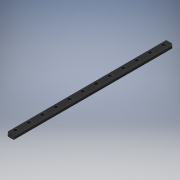
# Autodesk Inventor part: C-MLG9-235_r
Saved by Autodesk Inventor 2019 (Build 230136000, 136)
## iProperties
Created: 2023-08-25
Part Number: C-MLG9-235_r
Material: Generic
Catalog Web Link: www.cadenas.de
Description: C-MLG, C-MLGL, C-MLGB,C-GMLG, C-GMLGL_rail-Economy Miniature Liner guide - Standard type
Vendor: MISUMI
Document SubType Name: Modeling
Designer: psAdmin
Manufacturer: MISUMI
Mass: 11.5408 g
Surface Area: 89.2018 cm^2
Volume: 11.5408 cm^3
Density: 1 g/cm^3
Appearance: PSOLRGB-175-175-175
Category: PARTsolutions
Company: MISUMI
Title: C-MLG9-235
Author: Cadenas PARTsolutions
Comments: Economy Miniature Liner guide - Standard type
PSOL_IDENT_0: {$CADENAS_DATA/23d-libs/misumi/metric/06_linear_guides/c_mlg/c_mlg_rail.prj},209 {VTYP=3D},{NB=C-MLG
PSOL_IDENT_1: 9-235_r},{LINA=C-MLG9-235},{NN=C-MLG, C-MLGL, C-MLGB,C-GMLG, C-GMLGL_rail},{DATE=14.07.2023 05:43:34
PSOL_IDENT_2: },{GEOMDATE=01.12.2022 04:29:02},{VERSION=},{LINEID=20},{WBVAR=TS,ST,LT,L},{WBNUMERIC=L}  {NB=C-MLG9
PSOL_IDENT_3: -235_r},{LINA=C-MLG9-235},{KT=DUMMY},{PN=C-MLG9-235},{TS=},{ST=1},{LT=S},{LTALG='S', 'L Selectable T
PSOL_IDENT_4: ype', 'C', 'L Configurable Type'},{TYPE=C-MLG},{WR=9},{L=235},{LALG=[35,55,75,95,115,135,155,175,195
PSOL_IDENT_5: ,215,235,255,275]},{LALG1=[35,55,75,95,115,135,155,175,195,215,235,255,275]},{LALG2=[36:54/1],[56:74
PSOL_IDENT_6: /1],[76:94/1],[96:114/1],[116:134/1],[136:154/1],[156:174/1],[176:194/1],[196:214/1],[216:234/1],[23
PSOL_IDENT_7: 6:254/1],[256:274/1],[276:355/1]},{H=10},{H1=2.0},{N=5.5},{W=20},{B=15},{B1=2.5},{C=10},{L1=18.9},{L
PSOL_IDENT_8: 2=29.60},{GNN=Dia.1.4},{M=3},{LL=3.0},{ML=M3x3},{H2=1.8},{HRR=6.5},{D=6.0},{HH=3.5},{DD=3.5},{P=20},
PSOL_IDENT_9: {M1=12},{E=7.5},{NA=11},{R=1.00},{R1=0.400},{C1=0.30},{WR1=0.4},{WR2=0.92},{WR3=0.38},{HR1=4.5},{L3D=
PSOL_IDENT_10: 235.0},{LALG3=[35:355/1]}
NB: C-MLG9-235_r
NN: C-MLG, C-MLGL, C-MLGB,C-GMLG, C-GMLGL_rail
NT: Economy Miniature Liner guide - Standard type
NBSYN: $PN._r
LINA: C-MLG9-235
CATALOG: Misumi
PN: C-MLG9-235
TS: Assembly Products
ST: No Surface Treatment
LT: L Selectable Type
WR: 9
L: 235
H: 10
H1: 2
N: 5.5
W: 20
B: 15
B1: 2.5
C: 10
L1: 18.9
L2: 29.6
GNN: Dia.1.4
ML: M3x3
H2: 1.8
HRR: 6.5
D: 6
HH: 3.5
DD: 3.5
P: 20
E: 7.5
SUPPLIER: MISUMI
ARTICLENO: C-MLG9-235_r
BOMINFO: C-MLG9-235
CREATOR: CADENAS GmbH
Autodesk Inventor part; units mm, degrees
sketch "_____1" plane through (0, 0, 0) normal (0, 0, 1) x (1, 0, 0)
  line L0 (-4.5, 2.95) -> (-4.5, 2.1665)
  arc A0 (-3.9835, 1.65) -> (-4.5, 2.1665) centre (-4.9, 1.25) ccw
  line L1 (-3.9835, 1.65) -> (-3.6, 1.65)
  arc A1 (-3.6, 0.85) -> (-3.6, 1.65) centre (-3.6, 1.25) ccw
  line L2 (-3.6, 0.85) -> (-3.9835, 0.85)
  arc A2 (-4.5, 0.3335) -> (-3.9835, 0.85) centre (-4.9, 1.25) ccw
  line L3 (-4.5, 0.3335) -> (-4.5, -2.95)
  line L4 (-4.5, -2.95) -> (-4.2, -3.25)
  line L5 (-4.2, -3.25) -> (4.2, -3.25)
  line L6 (4.2, -3.25) -> (4.5, -2.95)
  line L7 (4.5, -2.95) -> (4.5, 0.3335)
  arc A3 (3.9835, 0.85) -> (4.5, 0.3335) centre (4.9, 1.25) ccw
  line L8 (3.9835, 0.85) -> (3.6, 0.85)
  arc A4 (3.6, 1.65) -> (3.6, 0.85) centre (3.6, 1.25) ccw
  line L9 (3.6, 1.65) -> (3.9835, 1.65)
  arc A5 (4.5, 2.1665) -> (3.9835, 1.65) centre (4.9, 1.25) ccw
  line L10 (4.5, 2.1665) -> (4.5, 2.95)
  line L11 (4.5, 2.95) -> (4.2, 3.25)
  line L12 (4.2, 3.25) -> (-4.2, 3.25)
  line L13 (-4.2, 3.25) -> (-4.5, 2.95)
  constraints: 28 end point, 12 point on circle, 6 centre point
extrude "Extrusion1" add sketch "_____1" along normal mid plane 235
sketch "_____5" plane through (0, 0, 110) normal (0, 0, 1) x (1, 0, 0)
  line L0 (0, 3.25) -> (0, -3.25)
  line L1 (0, -3.25) -> (-2.05, -3.25)
  line L2 (-2.05, -3.25) -> (-1.75, -2.95)
  line L3 (-1.75, -2.95) -> (-1.75, -0.25)
  line L4 (-1.75, -0.25) -> (-3, -0.25)
  line L5 (-3, -0.25) -> (-3, 2.95)
  line L6 (-3, 2.95) -> (-3.3, 3.25)
  line L7 (-3.3, 3.25) -> (0, 3.25)
  line L8 (0, 3.25) -> (0, -3.25)
  constraints: 18 end point
revolve "Revolution1" cut sketch "_____5" angle 360 about axis through (0, 3.25, 110) along (0, 1, 0)
pattern_linear "Rectangular Pattern1" count 12 spacing 20 along (0, 0, -1) of "Revolution1"
ref_plane "to_body_XY" through (0, -3.25, 0) normal (0, 0, 1) x (1, 0, 0)
ref_plane "to_body_YZ" through (0, -3.25, 0) normal (1, 0, 0) x (0, 1, 0)
ref_plane "to_body_ZX" through (0, -3.25, 0) normal (0, 1, 0) x (0, 0, 1)
body "Solid1"
